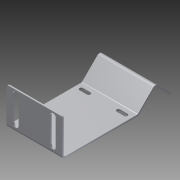
# Autodesk Inventor part: laserholder
Saved by Autodesk Inventor 2014 SP2 (Build 180246200, 246)
## iProperties
Created: 2016-05-15
Part Number: laserholder
Material: Aluminum 6061
Document SubType Name: Sheet Metal
Designer: cruiser
Density: 2.71 g/cm^3
Sheet Metal Rule: Default_mm
Appearance: Aluminum - Flat
Flat Pattern Width: 8.52185 cm
Flat Pattern Length: 3 cm
Flat Pattern Area: 25.5656 cm^2
Sheet Metal Width: 85.219 mm
Sheet Metal Length: 30.000 mm
Sheet Metal Area: 2556.556 mm^2
Mass: 5.55187 g
Surface Area: 54.2285 cm^2
Volume: 2.04866 cm^3
Author: cruiser
Autodesk Inventor part; units mm, degrees
ref_plane "YZ Plane" through (0, 0, 0) normal (1, 0, 0) x (0, 1, 0)
ref_plane "XZ Plane" through (0, 0, 0) normal (0, 1, 0) x (-1, 0, 0)
ref_plane "XY Plane" through (0, 0, 0) normal (0, 0, 1) x (1, 0, 0)
sketch "Sketch10" plane through (15, 0, 10) normal (1, 0, 0) x (0, 0, -1)
  line L0 (20, 0) -> (0, 0)
  line L1 (20, 0) -> (20, 0.7937)
  line L2 (0, 0) -> (0, 40.8076)
  line L3 (0, 40.8076) -> (-9.1924, 50)
  line L4 (0, 40.8076) -> (13, 40.8076) construction
  line L5 (-9.1924, 50) -> (0, 59.1924)
  point P0 (10, 0)
  dimension "d103" = 135
  dimension "d104" = 13
  dimension "d105" = 13
  dimension "d106" = 50
  measures "d103" angle of L4 L3
  measures "d104" distance of L3.end L5.end
  measures "d105" distance of L2.end L3.end
  measures "d106" distance from line of L0 L3.end
sketch "Sketch12" plane through (-15, 40.4788, 10) normal (0, 0, 1) x (1, 0, 0)
  line L0 (0, 0) -> (30, 0) projected
  line L1 (0, -38.8913) -> (0, 0) projected
  line L2 (15, -40.4788) -> (0, -40.4788)
  line L3 (0, -40.4788) -> (0, 0)
  line L4 (0, 0) -> (15, 0)
  line L5 (15, 0) -> (15, -40.4788)
  line L6 (3, -1.5875) -> (7, -1.5875) construction
  line L7 (3, -2.5875) -> (7, -2.5875)
  line L8 (7, -0.5875) -> (3, -0.5875)
  arc A0 (3, -0.5875) -> (3, -2.5875) centre (3, -1.5875) ccw
  arc A1 (7, -2.5875) -> (7, -0.5875) centre (7, -1.5875) ccw
  line L9 (27, -1.5875) -> (23, -1.5875) construction
  line L10 (27, -2.5875) -> (23, -2.5875)
  line L11 (23, -0.5875) -> (27, -0.5875)
  arc A2 (27, -2.5875) -> (27, -0.5875) centre (27, -1.5875) ccw
  arc A3 (23, -0.5875) -> (23, -2.5875) centre (23, -1.5875) ccw
  point P0 (5, -1.5875)
  point P1 (25, -1.5875)
  dimension "d116" = 2
  dimension "d117" = 2
  dimension "d118" = 1.5875
  dimension "d119" = 5
  constraints: 24 end point, 8 point on circle, 7 symmetric about line, 4 centre point, 4 parallel, 4 tangent, 1 horizontal, 1 midpoint, 1 perpendicular, 2 other
  measures "d116" distance of point (5, -1.588) L6.end
  measures "d117" diameter of A1
  measures "d118" distance between parallel lines of L4 L6
  measures "d119" distance from line of L1 point (5, -1.588)
sketch "Sketch13" plane through (0, 0, 0) normal (0, -1, 0) x (1, 0, 0)
  line L0 (15, 8.4125) -> (-15, 8.4125) projected
  line L1 (-15, 10) -> (-15, -10) projected
  line L2 (-15, -10) -> (15, -10) projected
  line L3 (15, -10) -> (15, 10) projected
  line L4 (0, 8.4125) -> (0, -10)
  line L5 (-15, -0.7937) -> (15, -0.7937)
  line L6 (-10, -6.2937) -> (-10, 4.7063) construction
  line L7 (-8.5, -6.2937) -> (-8.5, 4.7063)
  line L8 (-11.5, 4.7063) -> (-11.5, -6.2937)
  arc A0 (-11.5, -6.2937) -> (-8.5, -6.2937) centre (-10, -6.2937) ccw
  arc A1 (-8.5, 4.7063) -> (-11.5, 4.7063) centre (-10, 4.7063) ccw
  line L9 (10, -6.2937) -> (10, 4.7063) construction
  line L10 (8.5, -6.2937) -> (8.5, 4.7063)
  line L11 (11.5, 4.7063) -> (11.5, -6.2937)
  arc A2 (8.5, -6.2937) -> (11.5, -6.2937) centre (10, -6.2937) ccw
  arc A3 (11.5, 4.7063) -> (8.5, 4.7063) centre (10, 4.7063) ccw
  point P0 (0, 0)
  point P1 (-10, -0.7937)
  point P2 (10, -0.7937)
  dimension "d124" = 3
  dimension "d125" = 11
  dimension "d126" = 5
  constraints: 20 end point, 8 point on circle, 7 symmetric about line, 4 centre point, 4 tangent, 3 midpoint, 3 point on line, 1 parallel, 1 perpendicular, 2 other
  measures "d124" diameter of A1
  measures "d125" distance of L6.start L6.end
  measures "d126" distance between parallel lines of L1 L6
sketch "Sketch1" plane through (0, 0, 0) normal (0, 1, 0) x (-1, 0, 0)
  line L0 (15, -10) -> (-15, -10)
  line L1 (-15, -10) -> (-15, 10)
  line L2 (-15, 10) -> (15, 10)
  line L3 (15, 10) -> (15, -10)
  line L4 (15, -10) -> (-15, 10) construction
  line L5 (-15, -10) -> (15, 10) construction
  point P0 (0, 0)
  dimension "d10" = 30
  dimension "d11" = 20
  measures "d10" distance of L1.end L2.end
  measures "d11" distance of L0.end L1.end
extrude "Plate1" add sketch "Sketch1" along normal blind 0.7937
sketch "Sketch14" plane through (15, 0, 10) normal (1, 0, 0) x (0, 0, -1)
  line L0 (20, 0) -> (0, 0)
  line L1 (20, 0) -> (20, 0.7937)
  line L2 (20, 0) -> (20, 40.8076)
  line L3 (20, 40.8076) -> (10.8076, 50)
  line L4 (10.8076, 50) -> (20, 59.1924)
  point P0 (10, 0)
  dimension "d130" = 135
  dimension "d132" = 13
  dimension "d133" = 50
  dimension "d134" = 13
  measures "d130" angle of L3 L2
  measures "d132" distance of L3.end L4.end
  measures "d133" distance from line of L0 L3.end
  measures "d134" distance of L2.end L3.end
contour flange "Contour Flange6" sketch "Sketch14" thickness 0.7937 bend radius 0.7937 curves L2 L3 L4 edges at (0, 0.7937, -10) running between points at (15, 0.7937, -10) (-15, 0.7937, -10)
bend "Bend6"
corner "Corner6"
sketch "Sketch16" plane through (15, 40.15, -10) normal (0, 0, -1) x (-1, 0, 0)
  line L0 (0, 0) -> (30, 0) projected
  line L1 (0, -38.5625) -> (30, -38.5625) projected
  line L2 (15, 0) -> (15, -38.5625)
  line L3 (3, -3) -> (7, -3) construction
  line L4 (3, -4) -> (7, -4)
  line L5 (7, -2) -> (3, -2)
  arc A0 (3, -2) -> (3, -4) centre (3, -3) ccw
  arc A1 (7, -4) -> (7, -2) centre (7, -3) ccw
  line L6 (5, -3) -> (9, -3) construction
  line L7 (27, -3) -> (23, -3) construction
  line L8 (27, -4) -> (23, -4)
  line L9 (23, -2) -> (27, -2)
  arc A2 (27, -4) -> (27, -2) centre (27, -3) ccw
  arc A3 (23, -2) -> (23, -4) centre (23, -3) ccw
  line L10 (25, -3) -> (21, -3) construction
  point P0 (15, -40.15)
  dimension "d151" = 2
  dimension "d152" = 0
  dimension "d153" = 2
  dimension "d154" = 3
  dimension "d155" = 10
  constraints: 22 end point, 8 point on circle, 8 symmetric about line, 4 centre point, 4 tangent, 3 midpoint, 2 parallel, 1 collinear, 1 horizontal, 2 other
  measures "d151" distance of L6.start L3.end
  measures "d152" distance between parallel lines of L3 L6
  measures "d153" diameter of A1
  measures "d154" distance from line of L0 L6.start
  measures "d155" distance from line of L2 L6.start
extrude "Cut8" cut sketch "Sketch16" against normal blind 0.7937
sketch "Sketch15" plane through (0, 0, 0) normal (0, -1, 0) x (1, 0, 0)
  line L0 (15, -8.4125) -> (15, 10) projected
  line L1 (15, 10) -> (-15, 10) projected
  line L2 (-15, 10) -> (-15, -8.4125) projected
  line L3 (-15, 0.7938) -> (15, 0.7937)
  line L4 (-10, -6.1188) -> (-10, 7.7062) construction
  line L5 (-8.5, -6.1188) -> (-8.5, 7.7062)
  line L6 (-11.5, 7.7062) -> (-11.5, -6.1188)
  arc A0 (-11.5, -6.1188) -> (-8.5, -6.1188) centre (-10, -6.1188) ccw
  arc A1 (-8.5, 7.7062) -> (-11.5, 7.7062) centre (-10, 7.7062) ccw
  line L7 (0, 0.7938) -> (0, 10)
  line L8 (10, -6.1187) -> (10, 7.7062) construction
  line L9 (8.5, -6.1188) -> (8.5, 7.7062)
  line L10 (11.5, 7.7062) -> (11.5, -6.1188)
  arc A2 (8.5, -6.1188) -> (11.5, -6.1188) centre (10, -6.1187) ccw
  arc A3 (11.5, 7.7062) -> (8.5, 7.7062) centre (10, 7.7062) ccw
  point P0 (0, 0)
  point P1 (-10, 0.7937)
  point P2 (10, 0.7937)
  dimension "d144" = 3
  dimension "d146" = 5
  dimension "d147" = 13.825
  constraints: 20 end point, 8 point on circle, 7 symmetric about line, 5 midpoint, 4 centre point, 4 tangent, 1 parallel, 1 perpendicular, 1 point on line, 2 other
  measures "d144" diameter of A1
  measures "d146" distance between parallel lines of L2 L4
  measures "d147" distance of L4.start L4.end
extrude "Cut7" cut sketch "Sketch15" against normal blind 0.7937 contours L10 A2 L9 L3 | L3 L9 A3 L10 | L5 A0 L6 L3 | L3 L6 A1 L5
fillet "Corner Round3" radius 1 4 edges at (15, 0.3969, 10) (-15, 0.3969, 10) (15, 59.473, -9.7194) (-15, 59.473, -9.7194)
equation "\"BendRadius\" = Thickness"
equation "\"BendReliefWidth\" = Thickness"
equation "\"BendReliefDepth\" = 0.5 * Thickness"
equation "\"CornerReliefSize\" = 4 * Thickness"
equation "\"MinimumRemnant\" = 2 * Thickness"
equation "\"TransitionRadius\" = BendRadius"
equation "\"JacobiRadiusSize\" = BendRadius"
equation "\"GapSize\" = Thickness"
equation "\"d0\" = BendRadius"
equation "\"sm_thickness\" = 1.5875"
equation "\"very_thick_acrylic\" = 9.45"
equation "\"thick_acrylic\" = 5.88"
equation "\"thin_acrylic\" = 3.15"
equation "\"clear_acrylic\" = 3.15"
equation "\"wood_thickness\" = 6.72"
equation "\"m3_diameter\" = 3"
equation "\"m3_head\" = 6"
equation "\"m4_diameter\" = 4"
equation "\"m5_diameter\" = 5"
equation "\"m5_head\" = 10.3"
equation "\"brass_insert_drill\" = 4"
equation "\"m5_brass_insert_drill\" = 6.7"
equation "\"m3_press_nut_drill\" = 4.5"
equation "\"m5_press_nut_drill\" = 6.5"
equation "\"stepper_screw_space\" = 35"
equation "\"stepper_shaft_diameter\" = 5"
equation "\"stepper_body_diameter\" = 28"
equation "\"laser_body_diameter\" = 12"
equation "\"carrier_y\" = 251"
equation "\"carrier_z\" = 12"
equation "\"visor_x\" = 253.925"
equation "\"visor_y\" = 85.6"
equation "\"window_z\" = 332.225"
equation "\"window_y\" = 93.75"
equation "\"window_overlap\" = 48"
equation "\"acrylic_into_frame\" = 5"
equation "\"door_x\" = 251"
equation "\"door_z\" = 332.225"
equation "\"door_overlap\" = 48"
equation "\"reservoir_z\" = 35"
equation "\"linear_bearing_spacing\" = 209"
equation "\"tray_border\" = 25"
equation "\"bed_z\" = 25"
equation "\"crane_x\" = 234"
equation "\"crane_z2\" = 12"
equation "\"end_stop_spacing\" = 19"
equation "\"thumb_nut_offset_y\" = 0"
equation "\"thumb_nut_diameter\" = 7"
equation "\"z_min_from_center\" = 115"
equation "\"frame_top_z\" = 385"
equation "\"frame_bottom_z\" = 275"
equation "\"frame_total_z\" = 661.5875"
equation "\"frame_foot_z\" = 12"
equation "\"frame_tilt\" = 1deg"
equation "\"subframe_x\" = 66"
equation "\"subframe_y_offset\" = 27.5"
equation "\"laser_y_offset\" = 19.4"
equation "\"laser_diameter\" = 13"
equation "\"laser_z_offset\" = 55"
equation "\"laser_y\" = 15"
equation "\"laser_z\" = 75"
equation "\"t_galvo_frame\" = 6.72"
equation "\"galvo_frame_x\" = 66"
equation "\"galvo_frame_z\" = 85"
equation "\"galvo_frame_y_offset\" = 27.5"
equation "\"drawer_x\" = 202.02372"
equation "\"drawer_y\" = 72"
equation "\"drawer_support_from_top\" = 48"
equation "\"nema17_x\" = 43"
equation "\"laser_gap\" = 1"
equation "\"frame_screw_from_center\" = 25"
equation "\"drawer_screw_from_center\" = 55"
equation "\"frame_face_y\" = 45"
equation "\"switch_spacing\" = 19"
equation "\"subframe_y\" = 55"
equation "\"al_thickness\" = 1.5875"
equation "\"rivet_diameter\" = 3.3"
equation "\"bend_factor\" = 2.26205"
equation "\"al_bend\" = 3.591"
equation "\"sm_bend\" = 3.591"
equation "\"frame_x\" = 353.375"
equation "\"carrier_z2\" = 25"
equation "\"carrier_y2\" = 76.825"
equation "\"injection_plastic\" = 3.15"
equation "\"acrylic3_thickness\" = 3.15"
equation "\"laserresin\" = 5"
equation "\"al1_thickness\" = 0.79375"
equation "\"al2_bend\" = 3.591"
equation "\"acrylic2_thickness\" = 3.15"
equation "\"st1_bend\" = 2.06267"
equation "\"al3_thickness\" = 1.5875"
equation "\"al2_thickness\" = 1.5875"
equation "\"st2_thickness\" = 1.5875"
equation "\"st3_thickness\" = 1.5875"
equation "\"st3_bend\" = 3.591"
equation "\"al1_bend\" = 1.7955"
equation "\"frame_back_x\" = 278.2125"
equation "\"platform_upper_y\" = 46.625"
equation "\"frame_front_x\" = 280.23622"
equation "\"handle_d\" = 4.7625"
equation "\"platform_fold_x\" = 15"
equation "\"lmk8uu_z\" = 24"
equation "\"foot_t\" = 1.5875"
equation "\"crane_gap\" = 0.1"
equation "\"acrylic1_thickness\" = 5.88"
equation "\"foot_y\" = 194"
equation "\"al3_bend\" = 3.591"
equation "\"platform_t\" = 1.5875"
equation "\"handle_spacing\" = 50.8"
equation "\"platform_z\" = 65"
equation "\"nema17_shaft\" = 24"
equation "\"handle_projection\" = 20.6375"
equation "\"tray_to_platform_oversize\" = 0"
equation "\"frame_gap\" = 0.1"
equation "\"frame_front_t\" = 0.91186"
equation "\"foot_x\" = 192"
equation "\"lmk8uu_shaft\" = 15"
equation "\"shf8_y\" = 43"
equation "\"acme_nut_d\" = 19.1"
equation "\"platform_crane_gap\" = 0.1"
equation "\"Thickness\" = 0.79375"
body "Solid1"
